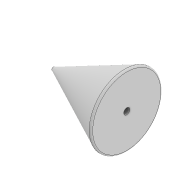
# Autodesk Inventor part: cone-fixed
Saved by Autodesk Inventor 2020 (Build 240168000, 168)
## iProperties
Created: 2021-06-07
Part Number: cone-fixed
Material: Generic
Document SubType Name: Modeling
Designer: Aidan Lee
Density: 1 g/cm^3
Appearance: Default
Author: Aidan Lee
Autodesk Inventor part; units mm, degrees
ref_plane "YZ Plane" through (0, 0, 0) normal (1, 0, 0) x (0, 1, 0)
ref_plane "XZ Plane" through (0, 0, 0) normal (0, 1, 0) x (-1, 0, 0)
ref_plane "XY Plane" through (0, 0, 0) normal (0, 0, 1) x (1, 0, 0)
sketch "Sketch1" plane through (0, 0, 0) normal (0, 0, 1) x (1, 0, 0)
  line L0 (0, 0) -> (0, 26.5512)
  line L1 (0, 26.5512) -> (-55.9167, 26.5512)
  line L2 (-55.9167, 26.5512) -> (0, 0)
  line L3 (-53.8107, 26.5512) -> (-53.8107, 25.5512)
  line L4 (-5, 26.5512) -> (-5, 2.3742)
  dimension "d15" = 1
  dimension "d16" = 5
  dimension "r" = 26.5512
  dimension "d18" = 25.4
  dimension "d19" = 48.8107
  constraints: 10 end point, 4 point on line, 3 vertical, 1 perpendicular
  measures "d15" distance of L3.start L3.end
  measures "d16" distance between parallel lines of L0 L4
  measures "r" distance of L0.start L0.end
  measures "d18" angle of L2 L1
  measures "d19" distance between parallel lines of L4 L3
revolve "Revolution1" add sketch "Sketch1" angle 360 about axis through (0, 26.5512, 0) along (-1, 0, 0) contours L2 L3 L1 L4
fillet "Fillet1" radius 1 1 edges at (-5, 50.7282, 0)
sketch "Sketch2" plane through (-5, 26.5512, 0) normal (1, 0, 0) x (0, 0, -1)
  circle A0 centre (0, 0) radius 2.05
  circle A1 centre (0, 0) radius 22.5952 projected
  point P0 (0, -26.5512)
  dimension "d7" = 4.1
  constraints: 1 centre point, 1 coincident
  measures "d7" diameter of A0
extrude "Extrusion1" cut sketch "Sketch2" against normal blind 15 contours A0
equation "\"d7\" = dowel + dowelgap"
equation "\"dowel\" = 4"
equation "\"dowelgap\" = 0.1"
body "Solid1"
